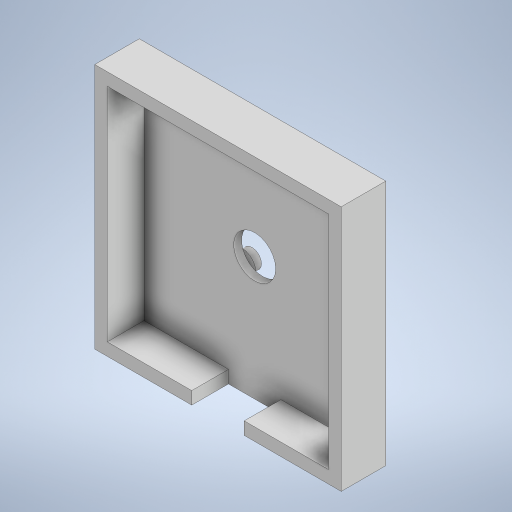
# Autodesk Inventor part: MagEncHolder
Saved by Autodesk Inventor 2024 (Build 280153000, 153)
## iProperties
Created: 2023-09-22
Part Number: MagEncHolder
Material: Generic
Document SubType Name: Modeling
Designer: RedStar
Density: 1 g/cm^3
Appearance: Default
Author: RedStar
Autodesk Inventor part; units mm, degrees
ref_plane "YZ Plane" through (0, 0, 0) normal (1, 0, 0) x (0, 1, 0)
ref_plane "XZ Plane" through (0, 0, 0) normal (0, 1, 0) x (-1, 0, 0)
ref_plane "XY Plane" through (0, 0, 0) normal (0, 0, 1) x (1, 0, 0)
sketch "Sketch1" plane through (0, 0, 0) normal (0, 0, 1) x (1, 0, 0)
  line L0 (-21.1, -21.1) -> (21.1, -21.1)
  line L1 (21.1, -21.1) -> (21.1, 21.1)
  line L2 (21.1, 21.1) -> (-21.1, 21.1)
  line L3 (-21.1, 21.1) -> (-21.1, -21.1)
  line L4 (-21.1, -21.1) -> (21.1, 21.1) construction
  line L5 (21.1, -21.1) -> (-21.1, 21.1) construction
  line L6 (-23.5, 23.5) -> (23.5, 23.5)
  line L7 (23.5, 23.5) -> (23.5, -23.5)
  line L8 (23.5, -23.5) -> (-23.5, -23.5)
  line L9 (-23.5, -23.5) -> (-23.5, 23.5)
  line L10 (-23.5, 23.5) -> (23.5, -23.5) construction
  line L11 (23.5, 23.5) -> (-23.5, -23.5) construction
  line L12 (-5, -21.1) -> (-5, -23.5)
  line L13 (5, -21.1) -> (5, -23.5)
  circle A0 centre (8, 8) radius 1.8
  circle A1 centre (8, -8) radius 1.8
  circle A2 centre (-8, -8) radius 1.8
  circle A3 centre (-8, 8) radius 1.8
  line L14 (-11, 11) -> (11, -11) construction
  line L15 (11, 11) -> (-11, -11) construction
  circle A4 centre (0, 0) radius 4
  circle A5 centre (-8, 8) radius 2.75
  circle A6 centre (-8, -8) radius 2.75
  circle A7 centre (8, 8) radius 2.75
  circle A8 centre (8, -8) radius 2.75
  dimension "d0" = 42.2
  dimension "d1" = 42.2
  dimension "d2" = 47
  dimension "d3" = 47
  dimension "d4" = 10
  dimension "d5" = 5
  dimension "d6" = 3.6
  dimension "d7" = 3.6
  dimension "d8" = 3.6
  dimension "d9" = 3.6
  dimension "d10" = 16
  dimension "d11" = 16
  dimension "d12" = 16
  dimension "d13" = 8
  dimension "d20" = 8
  dimension "d21" = 5.5
  dimension "d22" = 5.5
  dimension "d23" = 5.5
  dimension "d24" = 5.5
  constraints: 32 end point, 9 centre point, 8 point on line, 6 midpoint, 5 coincident, 4 parallel, 4 perpendicular, 2 horizontal
  measures "d0" distance of L2.end L1.end
  measures "d1" distance of L1.end L0.end
  measures "d2" distance of L7.end L8.end
  measures "d3" distance of L6.end L7.end
  measures "d4" distance between parallel lines of L13 L12
  measures "d5" distance from line of point (0, 0) L13
  measures "d6" diameter of A0
  measures "d7" diameter of A1
  measures "d8" diameter of A2
  measures "d9" diameter of A3
  measures "d10" distance of A2.centre A3.centre
  measures "d11" distance of A1.centre A0.centre
  measures "d12" distance of A0.centre A3.centre
  measures "d13" horizontal distance of point (0, 0) A3.centre
  measures "d20" diameter of A4
  measures "d21" diameter of A5
  measures "d22" diameter of A6
  measures "d23" diameter of A7
  measures "d24" diameter of A8
extrude "Extrusion1" add sketch "Sketch1" along normal blind 8.5 contours L0 L12 L8 L9 L6 L7 L13 L1 L2 L3
extrude "Extrusion2" add sketch "Sketch1" along normal blind 1.5 contours L3 L2 L1 L0 | L0 L13 L8 L12 | A0 | A1 | A2 | A3 | A5 | A6 | A7 | A8
extrude "Extrusion3" add sketch "Sketch1" against normal blind 4 contours A0 | A1 | A2 | A3 | A5 | A6 | A7 | A8
extrude "Extrusion4" add sketch "Sketch1" against normal blind 6 contours A0 | A1 | A2 | A3
body "Solid1"
